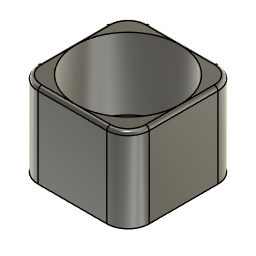
DrinkMixerV1CupAdapter (Autodesk Fusion 360 design; units mm, degrees)
Autodesk Fusion 360 part; units mm, degrees
note: some values were not read from the file. Set by a fixed rule: which sketch regions a step uses.
sketch "Sketch1" plane through (0, 0, 0) normal (0, 0, 1) x (1, 0, 0)
  line L0 (39.37, 39.37) -> (-39.37, 39.37)
  line L1 (-39.37, 39.37) -> (-39.37, -39.37)
  line L2 (-39.37, -39.37) -> (39.37, -39.37)
  line L3 (39.37, -39.37) -> (39.37, 39.37)
  line L4 (39.37, 39.37) -> (-39.37, -39.37) construction
  line L5 (-39.37, 39.37) -> (39.37, -39.37) construction
  dimension "d9" = 78.74
  dimension "d10" = 78.74
  constraint horizontal L0
  constraint perpendicular L0 L1
  constraint parallel L0 L2
  constraint parallel L1 L3
  constraint coincident L4 origin
  constraint coincident L5 origin
  measures "d9" distance of L1.end L2.end
  measures "d10" distance of L0.end L1.end
extrude "Extrude1" add sketch "Sketch1" along normal blind 50.8
sketch "Sketch2" plane through (0, 0, 50.8) normal (0, 0, 1) x (-1, 0, 0)
  line L0 (-39.37, 39.37) -> (-39.37, -39.37)
  line L1 (-39.37, -39.37) -> (39.37, -39.37)
  line L2 (39.37, -39.37) -> (39.37, 39.37)
  line L3 (39.37, 39.37) -> (-39.37, 39.37)
  circle A0 centre (0, 0) radius 36.83
  dimension "d13" = 73.66
  constraint coincident A0.centre origin
  measures "d13" diameter of A0
extrude "Extrude2" cut sketch "Sketch2" against normal up to surface (50.8 mm away) contours A0
sketch "Sketch3" plane through (0, 0, 0) normal (0, 0, -1) x (1, 0, 0)
  circle A0 centre (0, 0) radius 36.83
  line L0 (39.37, -39.37) -> (39.37, 39.37)
  line L1 (39.37, 39.37) -> (-39.37, 39.37)
  line L2 (-39.37, 39.37) -> (-39.37, -39.37)
  line L3 (-39.37, -39.37) -> (39.37, -39.37)
  line L4 (-39.37, 39.37) -> (39.37, 39.37)
  line L5 (39.37, 39.37) -> (39.37, -39.37)
  line L6 (39.37, -39.37) -> (-39.37, -39.37)
  line L7 (-39.37, -39.37) -> (-39.37, 39.37)
  constraint horizontal L4
  constraint vertical L5
  constraint horizontal L6
  constraint vertical L7
  constraint coincident L0.start L3.end
  constraint coincident L1.end L2.start
extrude "Extrude3" add sketch "Sketch3" along normal blind 2.54 contours A0 | L0 L1 L2 L3 L4 L5 L6 L7
sketch "Sketch4" plane through (0, 0, -2.54) normal (0, 0, -1) x (1, 0, 0)
  line L0 (-39.37, -39.37) -> (39.37, -39.37)
  line L1 (39.37, -39.37) -> (39.37, 39.37)
  line L2 (39.37, 39.37) -> (-39.37, 39.37)
  line L3 (-39.37, 39.37) -> (-39.37, -39.37)
  line L4 (-20.32, 26.035) -> (20.32, 26.035)
  line L5 (20.32, 26.035) -> (20.32, -26.035)
  line L6 (20.32, -26.035) -> (-20.32, -26.035)
  line L7 (-20.32, -26.035) -> (-20.32, 26.035)
  line L8 (-20.32, 26.035) -> (20.32, -26.035) construction
  line L9 (20.32, 26.035) -> (-20.32, -26.035) construction
  dimension "d18" = 40.64
  dimension "d19" = 52.07
  constraint horizontal L4
  constraint perpendicular L4 L5
  constraint parallel L4 L6
  constraint parallel L5 L7
  constraint coincident L8 origin
  constraint coincident L9 origin
  measures "d18" distance of L5.end L6.end
  measures "d19" distance of L4.end L5.end
extrude "Extrude4" add sketch "Sketch4" along normal blind 5.7912 contours L4 L5 L6 L7
sketch "Sketch5" plane through (0, 0, -8.3312) normal (0, 0, -1) x (1, 0, 0)
  line L0 (-20.32, -26.035) -> (20.32, -26.035)
  line L1 (20.32, -26.035) -> (20.32, 26.035)
  line L2 (20.32, 26.035) -> (-20.32, 26.035)
  line L3 (-20.32, 26.035) -> (-20.32, -26.035)
  line L4 (-12.065, 20.32) -> (12.065, 20.32)
  line L5 (12.065, 20.32) -> (12.065, -20.32)
  line L6 (12.065, -20.32) -> (-12.065, -20.32)
  line L7 (-12.065, -20.32) -> (-12.065, 20.32)
  line L8 (-12.065, 20.32) -> (12.065, -20.32) construction
  line L9 (12.065, 20.32) -> (-12.065, -20.32) construction
  circle A0 centre (12.065, -20.32) radius 2.4765
  circle A1 centre (-12.065, -20.32) radius 2.4765
  circle A2 centre (-12.065, 20.32) radius 2.4765
  circle A3 centre (12.065, 20.32) radius 2.4765
  dimension "d23" = 24.13
  dimension "d24" = 40.64
  dimension "d26" = 4.953
  dimension "d27" = 4.953
  dimension "d28" = 4.953
  dimension "d29" = 4.953
  constraint horizontal L4
  constraint perpendicular L4 L5
  constraint parallel L4 L6
  constraint parallel L5 L7
  constraint coincident L8 origin
  constraint coincident L9 origin
  constraint coincident L5.end L6.start
  constraint coincident L6.end L7.start
  constraint coincident L4.start L7.end
  constraint coincident L4.end L5.start
  measures "d23" distance of L5.end L6.end
  measures "d24" distance of L4.end L5.end
  measures "d26" diameter of A0
  measures "d27" diameter of A1
  measures "d28" diameter of A2
  measures "d29" diameter of A3
extrude "Extrude5" cut sketch "Sketch5" against normal up to surface (59.1312 mm away) contours L4 L7 A2 | L4 L7 A2 | L4 L5 A3 | L4 L5 A3 | L6 L7 A1 | L6 L7 A1 | L5 L6 A0 | L5 L6 A0
sketch "Sketch6" plane through (0, 0, 0) normal (0, 0, 1) x (-1, 0, 0)
  circle A0 centre (12.065, -20.32) radius 2.4765
  circle A1 centre (12.065, 20.32) radius 2.4765
  circle A2 centre (-12.065, -20.32) radius 2.4765
  circle A3 centre (-12.065, 20.32) radius 2.4765
  circle A4 centre (0, 0) radius 36.83
  line L0 (-12.065, 20.32) -> (12.065, 20.32)
  line L1 (12.065, 20.32) -> (12.065, -20.32)
  line L2 (12.065, -20.32) -> (-12.065, -20.32)
  line L3 (-12.065, -20.32) -> (-12.065, 20.32)
  circle A5 centre (-12.065, 20.32) radius 4.445
  circle A6 centre (12.065, 20.32) radius 4.445
  circle A7 centre (-12.065, -20.32) radius 4.445
  circle A8 centre (12.065, -20.32) radius 4.445
  dimension "d33" = 8.89
  dimension "d34" = 8.89
  dimension "d35" = 8.89
  dimension "d36" = 8.89
  constraint horizontal L0
  constraint vertical L1
  constraint horizontal L2
  constraint vertical L3
  constraint coincident A0.centre L1.end
  constraint coincident A3.centre L0.start
  constraint coincident A1.centre L0.end
  constraint coincident A2.centre L2.end
  measures "d33" diameter of A5
  measures "d34" diameter of A6
  measures "d35" diameter of A7
  measures "d36" diameter of A8
extrude "Extrude6" add sketch "Sketch6" along normal blind 6.35 contours L0 L1 L2 L3 A5 A6 A7 A8 | A4
extrude "Extrude7" add 1 faces at (29.7771, -31.0719, 50.8) along direction (0, 0, 1) blind 6.35
fillet "Fillet1" radius 15 4 edges at (39.37, -39.37, 27.305) (39.37, 39.37, 27.305) (-39.37, -39.37, 27.305) (-39.37, 39.37, 27.305)
fillet "Fillet2" radius 2.5 8 edges at (-34.9766, 34.9766, 57.15) (-39.37, 0, 57.15) (-34.9766, -34.9766, 57.15) (0, -39.37, 57.15) (34.9766, -34.9766, 57.15) (39.37, 0, 57.15) (34.9766, 34.9766, 57.15) (0, 39.37, 57.15)
equation "CupBaseDiameter = 2.7 in"
equation "CupHeight = 2 in"
equation "CupTopDiameter = 2.9 in"
equation "HoleDistanceLength = 0.95 in"
equation "HoleDistanceWidth = 1.6 in"
equation "BaseLength = 1.6 in"
equation "BaseWidth = 2.05 in"
equation "CupTop = CupTopDiameter + 0.2 in"
equation "d9 = CupTop"
equation "d10 = CupTop"
equation "d11 = CupHeight"
equation "d13 = CupTopDiameter"
equation "d18 = BaseLength"
equation "d19 = BaseWidth"
equation "BaseHeight = 0.228 in"
equation "d21 = BaseHeight"
equation "d23 = HoleDistanceLength"
equation "d24 = HoleDistanceWidth"
equation "ScrewHoleDiameter = 0.195 in"
equation "d26 = ScrewHoleDiameter"
equation "d27 = ScrewHoleDiameter"
equation "d28 = ScrewHoleDiameter"
equation "d29 = ScrewHoleDiameter"
equation "ScrewTopDiamater = 0.35 in"
equation "d33 = ScrewTopDiamater"
equation "d34 = ScrewTopDiamater"
equation "d35 = ScrewTopDiamater"
equation "d36 = ScrewTopDiamater"
